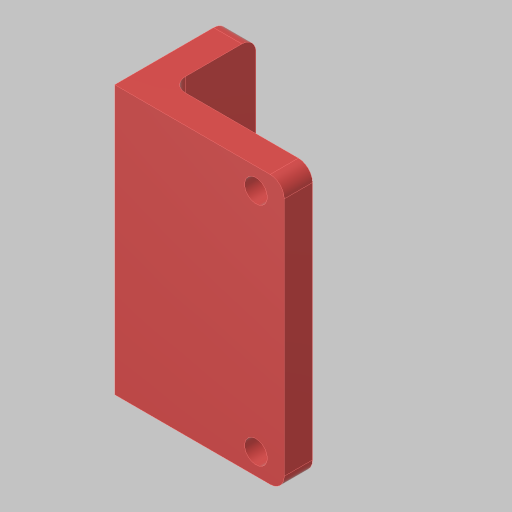
# Autodesk Inventor part: HS-001
Saved by Autodesk Inventor 2023.5 (Build 275446000, 446)
## iProperties
Created: 2025-02-22
Part Number: HS-001
Material: ABS Plastic
Document SubType Name: Modeling
Designer: slick
Density: 1.06 g/cm^3
Appearance: Smooth - Red
Author: slick
Autodesk Inventor part; units mm, degrees
ref_plane "YZ Plane" through (0, 0, 0) normal (1, 0, 0) x (0, 1, 0)
ref_plane "XZ Plane" through (0, 0, 0) normal (0, 1, 0) x (-1, 0, 0)
ref_plane "XY Plane" through (0, 0, 0) normal (0, 0, 1) x (1, 0, 0)
sketch "Sketch1" plane through (0, 0, 0) normal (0, 1, 0) x (-1, 0, 0)
  line L0 (0, 0) -> (0, -6.35)
  line L1 (0, -6.35) -> (31.75, -6.35)
  line L2 (31.75, -6.35) -> (31.75, -25.4)
  line L3 (31.75, -25.4) -> (38.1, -25.4)
  line L4 (38.1, -25.4) -> (38.1, 0)
  line L5 (38.1, 0) -> (0, 0)
  dimension "d0" = 6.35
  dimension "d1" = 38.1
  dimension "d2" = 25.4
  constraints: 12 end point, 6 perpendicular, 1 vertical
  measures "d0" distance of L0.start L0.end
  measures "d1" distance of L4.end L0.start
  measures "d2" distance of L3.end L4.end
extrude "Extrusion1" add sketch "Sketch1" along normal blind 60.325
sketch "Sketch2" plane through (-38.1, 0, 0) normal (0, 0, 1) x (1, 0, 0)
  line L0 (31.75, 4.7625) -> (31.75, 55.5625) construction
  line L1 (38.1, 0) -> (38.1, 60.325) construction
  point P0 (31.75, 30.1625)
  point P1 (38.1, 30.1625)
  dimension "d5" = 50.8
  dimension "d6" = 6.35
  constraints: 2 end point, 2 midpoint, 1 horizontal alignment, 1 vertical
  measures "d5" distance of L0.start L0.end
  measures "d6" distance between parallel lines of L1 L0
hole "Hole1" at (-6.35, 4.7625, 0) at (-6.35, 55.5625, 0) direction (0, 0, -1) diameter 5.1054 end through all clearance for "Flat Head Machine Screw (82)" size "#10" standard "Ansi Unified Screw Threads"
sketch "Sketch3" plane through (-38.1, 0, -25.4) normal (-1, 0, 0) x (0, 0, 1)
  line L0 (12.7, 46.1625) -> (12.7, 14.1625) construction
  line L1 (0, 0) -> (0, 60.325) construction
  line L2 (0, 60.325) -> (25.4, 60.325) construction
  point P0 (25.4, 0)
  point P1 (12.7, 30.1625)
  point P2 (0, 30.1625)
  point P3 (12.7, 60.325)
  dimension "d14" = 32
  constraints: 3 midpoint, 2 end point, 1 horizontal alignment, 1 vertical, 1 vertical alignment
  measures "d14" distance of L0.start L0.end
hole "Hole2" at (-38.1, 46.1625, -12.7) at (-38.1, 14.1625, -12.7) direction (1, 0, 0) diameter 3.81 end through all clearance for "Flat Head Machine Screw (82)" size "#6" standard "Ansi Unified Screw Threads"
fillet "Fillet1" radius 3.175 5 edges at (-31.75, 30.1625, -6.35) (-34.925, 60.325, -25.4) (-34.925, 0, -25.4) (0, 0, -3.175) (0, 60.325, -3.175)
body "Solid1"
